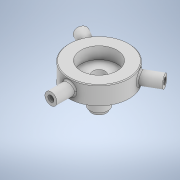
# Autodesk Inventor part: Ch4 Part 2
Saved by Autodesk Inventor 2020 (Build 240168000, 168)
## iProperties
Created: 2021-02-11
Part Number: Ch4 Part 2
Material: Generic
Document SubType Name: Modeling
Designer: austi
Density: 1 g/cm^3
Appearance: Default
Author: austi
Autodesk Inventor part; units mm, degrees
ref_plane "YZ Plane" through (0, 0, 0) normal (1, 0, 0) x (0, 1, 0)
ref_plane "XZ Plane" through (0, 0, 0) normal (0, 1, 0) x (-1, 0, 0)
ref_plane "XY Plane" through (0, 0, 0) normal (0, 0, 1) x (1, 0, 0)
sketch "Sketch1" plane through (0, 0, 0) normal (0, 1, 0) x (-1, 0, 0)
  circle A0 centre (0, 0) radius 31.75
  dimension "d0" = 63.5
  constraints: 1 centre point, 1 coincident
  measures "d0" diameter of A0
extrude "Extrusion1" add sketch "Sketch1" along normal blind 19.05
sketch "Sketch2" plane through (0, 0, 0) normal (0, 0, 1) x (1, 0, 0)
  line L0 (-44.45, 0) -> (44.45, 0) projected
  line L1 (0, -3.81) -> (0, 22.86) projected
  circle A0 centre (0, 9.525) radius 6.35
  point P0 (0, 0)
  dimension "d3" = 12.7
  constraints: 1 centre point, 1 midpoint
  measures "d3" diameter of A0
extrude "Extrusion2" add sketch "Sketch2" along normal blind 50.8
pattern_circular "Circular Pattern1" count 3 over 360 about axis through (0, -10, 0) along (0, 1, 0) of "Extrusion2"
sketch "Sketch3" plane through (0, 19.05, 0) normal (0, 1, 0) x (1, 0, 0)
  point P0 (0, 0)
  point P1 (0, 0)
  constraints: 1 coincident
hole "Hole1" at (0, 19.05, 0) direction (0, -1, 0) diameter 9.525 end through all counterbore diameter 38.1 counterbore depth 12.7
sketch "Sketch4" plane through (0, 9.525, 50.8) normal (0, 0, 1) x (1, 0, 0)
  circle A0 centre (0, 0) radius 6.35 projected
  point P0 (0, -9.525)
  constraints: 2 coincident
hole "Hole2" at (0, 9.525, 50.8) direction (0, 0, -1) diameter 6.4008 depth 25.4 tip angle 118 thread size "5/16-18 UNC" class "2B" standard "ANSI Unified Screw Threads"
pattern_circular "Circular Pattern2" count 3 over 360 about axis through (0, -10, 0) along (0, 1, 0) of "Hole2"
sketch "Sketch5" plane through (0, 0, 0) normal (0, -1, 0) x (1, 0, 0)
  circle A0 centre (0, 0) radius 9.525
  dimension "d26" = 19.05
  constraints: 1 centre point, 1 coincident
  measures "d26" diameter of A0
extrude "Extrusion3" add sketch "Sketch5" along normal blind 25.4
sketch "Sketch6" plane through (0, 0, 0) normal (0, 1, 0) x (1, 0, 0)
  circle A0 centre (0, 0) radius 31.75 projected
  constraints: 1 coincident
hole "Hole3" at (0, 0, 0) direction (0, -1, 0) diameter 12.7 end through all both
sketch "Sketch7" plane through (0, 0, 0) normal (0, -1, 0) x (1, 0, 0)
  point P0 (0, 0)
chamfer "Chamfer1" distance 3.302 angle 30 1 edges at (-9.525, -25.4, 0) measured on face at (-9.525, -24.9, 0)
chamfer "Chamfer2" distance 0.7937 angle 45 1 edges at (31.75, 19.05, 0) measured on face at (31.25, 19.05, 0)
fillet "Fillet1" radius 1.5875 3 edges at (30.1158, 9.5273, -10.055) (-23.7658, 9.5273, -21.0535) (-6.35, 9.5273, 31.1085)
body "Solid1"
